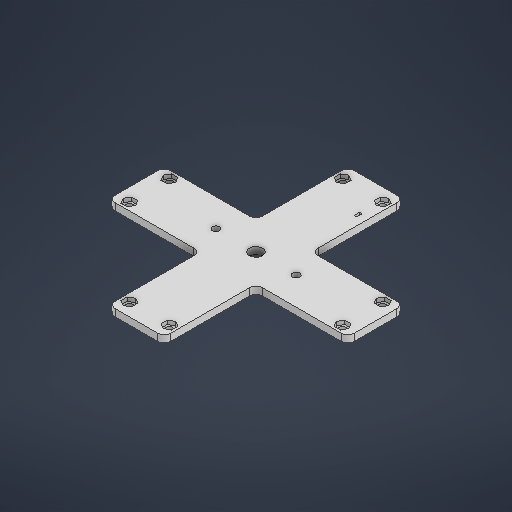
# Autodesk Inventor part: motor_holder
Saved by Autodesk Inventor 2026 (Build 300175050, 175E)
## iProperties
Created: 2025-01-16
Part Number: motor_holder
Material: Generic
Document SubType Name: Modeling
Designer: aduwa
Density: 1 g/cm^3
Appearance: Default
Author: aduwa
Autodesk Inventor part; units mm, degrees
ref_plane "YZ Plane" through (0, 0, 0) normal (1, 0, 0) x (0, 1, 0)
ref_plane "XZ Plane" through (0, 0, 0) normal (0, 1, 0) x (-1, 0, 0)
ref_plane "XY Plane" through (0, 0, 0) normal (0, 0, 1) x (1, 0, 0)
sketch "Sketch1" plane through (0, 0, 0) normal (0, 1, 0) x (1, 0, 0)
  circle A0 centre (0, 0) radius 2.25
  circle A1 centre (31, 0) radius 2.25
  circle A2 centre (0, 31) radius 2.25
  circle A3 centre (31, 31) radius 2.25
  circle A4 centre (15.5, 15.5) radius 5.125
  line L0 (-6, 37) -> (37, 37)
  line L1 (37, 37) -> (37, -6)
  line L2 (37, -6) -> (-6, -6)
  line L3 (-6, -6) -> (-6, 37)
  line L4 (-6, 37) -> (37, -6) construction
  line L5 (37, 37) -> (-6, -6) construction
  line L6 (-6, -6) -> (37, -6)
  circle A5 centre (0, 98) radius 2.75
  circle A6 centre (31, 98) radius 2.75
  line L7 (-6, 37) -> (37, 37)
  line L8 (37, 37) -> (37, 108)
  line L9 (37, 108) -> (-6, 108)
  line L10 (-6, 108) -> (-6, 37)
  line L11 (15.5, 15.5) -> (22.827, 15.5)
  line L12 (13, 103) -> (18, 103)
  line L13 (15.5, 103) -> (15.5, 96.4439)
  arc A7 (0, 95.25) -> (0, 100.75) centre (0, 98) ccw
  circle A8 centre (-15.5, 15.5) radius 2.7971
  circle A9 centre (46.5, 15.5) radius 2.7971
  line L14 (0, 93.4736) -> (-3.92, 95.7368)
  line L15 (-3.92, 95.7368) -> (-3.92, 100.2632)
  line L16 (-3.92, 100.2632) -> (0, 102.5264)
  line L17 (0, 102.5264) -> (3.92, 100.2632)
  line L18 (3.92, 100.2632) -> (3.92, 95.7368)
  line L19 (3.92, 95.7368) -> (0, 93.4736)
  line L20 (4.17, 100.4076) -> (0, 102.8151)
  line L21 (0, 102.8151) -> (-4.17, 100.4076)
  line L22 (-4.17, 100.4076) -> (-4.17, 95.5924)
  line L23 (-4.17, 95.5924) -> (0, 93.1849)
  line L24 (0, 93.1849) -> (4.17, 95.5924)
  line L25 (4.17, 95.5924) -> (4.17, 100.4076)
  circle A10 centre (31, 98) radius 2.75
  circle A11 centre (31, 98) radius 2.75
  arc A12 (31, 100.75) -> (31, 95.25) centre (31, 98) ccw
  line L26 (31, 93.4736) -> (34.92, 95.7368)
  line L27 (34.92, 95.7368) -> (34.92, 100.2632)
  line L28 (34.92, 100.2632) -> (31, 102.5264)
  line L29 (31, 102.5264) -> (27.08, 100.2632)
  line L30 (27.08, 100.2632) -> (27.08, 95.7368)
  line L31 (27.08, 95.7368) -> (31, 93.4736)
  line L32 (26.83, 100.4076) -> (31, 102.8151)
  line L33 (31, 102.8151) -> (35.17, 100.4076)
  line L34 (35.17, 100.4076) -> (35.17, 95.5924)
  line L35 (35.17, 95.5924) -> (31, 93.1849)
  line L36 (31, 93.1849) -> (26.83, 95.5924)
  line L37 (26.83, 95.5924) -> (26.83, 100.4076)
  line L38 (-64.7368, -3.92) -> (-69.2632, -3.92)
  line L39 (-69.4076, -4.17) -> (-64.5924, -4.17)
  line L40 (-69.2632, -3.92) -> (-71.5264, 0)
  line L41 (-71.8151, 0) -> (-69.4076, -4.17)
  circle A13 centre (-67, 31) radius 2.75
  line L42 (-72, 13) -> (-72, 18)
  line L43 (-69.2632, 27.08) -> (-64.7368, 27.08)
  line L44 (-64.7368, 34.92) -> (-69.2632, 34.92)
  line L45 (-64.5924, 26.83) -> (-69.4076, 26.83)
  circle A14 centre (-67, 31) radius 2.75
  circle A15 centre (-67, 31) radius 2.75
  arc A16 (-69.75, 31) -> (-64.25, 31) centre (-67, 31) ccw
  line L46 (-72, 15.5) -> (-65.4439, 15.5)
  line L47 (-69.2632, 34.92) -> (-71.5264, 31)
  line L48 (-71.8151, 31) -> (-69.4076, 35.17)
  line L49 (-69.4076, 35.17) -> (-64.5924, 35.17)
  line L50 (-71.5264, 31) -> (-69.2632, 27.08)
  line L51 (-69.4076, 26.83) -> (-71.8151, 31)
  line L52 (-62.4736, 0) -> (-64.7368, -3.92)
  line L53 (-64.5924, -4.17) -> (-62.1849, 0)
  circle A17 centre (-67, 0) radius 2.75
  arc A18 (-64.25, 0) -> (-69.75, 0) centre (-67, 0) ccw
  line L54 (-71.5264, 0) -> (-69.2632, 3.92)
  line L55 (-69.4076, 4.17) -> (-71.8151, 0)
  line L56 (-69.2632, 3.92) -> (-64.7368, 3.92)
  line L57 (-64.5924, 4.17) -> (-69.4076, 4.17)
  line L58 (-62.1849, 0) -> (-64.5924, 4.17)
  line L59 (-64.7368, 3.92) -> (-62.4736, 0)
  line L60 (-62.1849, 31) -> (-64.5924, 26.83)
  line L61 (-64.7368, 27.08) -> (-62.4736, 31)
  line L62 (-77, -6) -> (-6, -6)
  line L63 (-62.4736, 31) -> (-64.7368, 34.92)
  line L64 (-64.5924, 35.17) -> (-62.1849, 31)
  line L65 (-77, 37) -> (-77, -6)
  line L66 (-6, 37) -> (-77, 37)
  line L67 (34.92, -64.7368) -> (34.92, -69.2632)
  line L68 (35.17, -69.4076) -> (35.17, -64.5924)
  line L69 (34.92, -69.2632) -> (31, -71.5264)
  line L70 (31, -71.8151) -> (35.17, -69.4076)
  circle A19 centre (0, -67) radius 2.75
  line L71 (18, -72) -> (13, -72)
  line L72 (3.92, -69.2632) -> (3.92, -64.7368)
  line L73 (-3.92, -64.7368) -> (-3.92, -69.2632)
  line L74 (4.17, -64.5924) -> (4.17, -69.4076)
  circle A20 centre (0, -67) radius 2.75
  circle A21 centre (0, -67) radius 2.75
  arc A22 (0, -69.75) -> (0, -64.25) centre (0, -67) ccw
  line L75 (15.5, -72) -> (15.5, -65.4439)
  line L76 (-3.92, -69.2632) -> (0, -71.5264)
  line L77 (0, -71.8151) -> (-4.17, -69.4076)
  line L78 (-4.17, -69.4076) -> (-4.17, -64.5924)
  line L79 (0, -71.5264) -> (3.92, -69.2632)
  line L80 (4.17, -69.4076) -> (0, -71.8151)
  line L81 (31, -62.4736) -> (34.92, -64.7368)
  line L82 (35.17, -64.5924) -> (31, -62.1849)
  circle A23 centre (31, -67) radius 2.75
  arc A24 (31, -64.25) -> (31, -69.75) centre (31, -67) ccw
  line L83 (31, -71.5264) -> (27.08, -69.2632)
  line L84 (26.83, -69.4076) -> (31, -71.8151)
  line L85 (27.08, -69.2632) -> (27.08, -64.7368)
  line L86 (26.83, -64.5924) -> (26.83, -69.4076)
  line L87 (31, -62.1849) -> (26.83, -64.5924)
  line L88 (27.08, -64.7368) -> (31, -62.4736)
  line L89 (0, -62.1849) -> (4.17, -64.5924)
  line L90 (3.92, -64.7368) -> (0, -62.4736)
  line L91 (37, -77) -> (37, -6)
  line L92 (0, -62.4736) -> (-3.92, -64.7368)
  line L93 (-4.17, -64.5924) -> (0, -62.1849)
  line L94 (-6, -77) -> (37, -77)
  line L95 (-6, -6) -> (-6, -77)
  line L96 (95.7368, 34.92) -> (100.2632, 34.92)
  line L97 (100.4076, 35.17) -> (95.5924, 35.17)
  line L98 (100.2632, 34.92) -> (102.5264, 31)
  line L99 (102.8151, 31) -> (100.4076, 35.17)
  circle A25 centre (98, 0) radius 2.75
  line L100 (103, 18) -> (103, 13)
  line L101 (100.2632, 3.92) -> (95.7368, 3.92)
  line L102 (95.7368, -3.92) -> (100.2632, -3.92)
  line L103 (95.5924, 4.17) -> (100.4076, 4.17)
  circle A26 centre (98, 0) radius 2.75
  circle A27 centre (98, 0) radius 2.75
  arc A28 (100.75, 0) -> (95.25, 0) centre (98, 0) ccw
  line L104 (103, 15.5) -> (96.4439, 15.5)
  line L105 (100.2632, -3.92) -> (102.5264, 0)
  line L106 (102.8151, 0) -> (100.4076, -4.17)
  line L107 (100.4076, -4.17) -> (95.5924, -4.17)
  line L108 (102.5264, 0) -> (100.2632, 3.92)
  line L109 (100.4076, 4.17) -> (102.8151, 0)
  line L110 (93.4736, 31) -> (95.7368, 34.92)
  line L111 (95.5924, 35.17) -> (93.1849, 31)
  circle A29 centre (98, 31) radius 2.75
  arc A30 (95.25, 31) -> (100.75, 31) centre (98, 31) ccw
  line L112 (102.5264, 31) -> (100.2632, 27.08)
  line L113 (100.4076, 26.83) -> (102.8151, 31)
  line L114 (100.2632, 27.08) -> (95.7368, 27.08)
  line L115 (95.5924, 26.83) -> (100.4076, 26.83)
  line L116 (93.1849, 31) -> (95.5924, 26.83)
  line L117 (95.7368, 27.08) -> (93.4736, 31)
  line L118 (93.1849, 0) -> (95.5924, 4.17)
  line L119 (95.7368, 3.92) -> (93.4736, 0)
  line L120 (108, 37) -> (37, 37)
  line L121 (93.4736, 0) -> (95.7368, -3.92)
  line L122 (95.5924, -4.17) -> (93.1849, 0)
  line L123 (108, -6) -> (108, 37)
  line L124 (37, -6) -> (108, -6)
  point P0 (37, 37)
  point P1 (37, 37)
  point P2 (-3.5, 98)
  point P3 (34.5, 98)
  point P4 (-67, -3.5)
  point P5 (-67, 34.5)
  point P6 (34.5, -67)
  point P7 (-3.5, -67)
  point P8 (98, 34.5)
  point P9 (98, -3.5)
  point P10 (-6, -6)
  point P11 (-6, -6)
  point P12 (-6, -6)
  point P13 (-6, -6)
  point P14 (-6, -6)
  point P15 (37, 37)
  dimension "d3" = 4.5
  dimension "d5" = 31
  dimension "d6" = 10.25
  dimension "d8" = 43
  dimension "d23" = 5.5
  dimension "d24" = 31
  dimension "d25" = 31
  dimension "d27" = 6
  dimension "d28" = 10
  dimension "d71" = 62
  dimension "d72" = 31
  dimension "d73" = 7.84
  dimension "d74" = 0.25
  dimension "d81" = 82.5
  dimension "d84" = 360
  constraints: 250 end point, 31 centre point, 17 symmetric about line, 16 point on circle, 12 coincident, 6 equal radius, 5 horizontal, 4 parallel, 3 horizontal alignment, 3 midpoint, 2 perpendicular, 2 vertical alignment, 1 point on line, 1 vertical, 341 other
  measures "d3" diameter of A0
  measures "d5" distance of A0.centre A2.centre
  measures "d6" diameter of A4
  measures "d8" distance of L0.end L1.end
  measures "d23" diameter of A5
  measures "d24" distance of A6.centre A5.centre
  measures "d25" distance of A1.centre A0.centre
  measures "d27" distance from line of L0 A2.centre
  measures "d28" distance from line of L9 A5.centre
  measures "d71" distance of A9.centre A8.centre
  measures "d72" distance of L11.start A8.centre
  measures "d73" distance between parallel lines of L15 L18
  measures "d74" distance between parallel lines of L17 L20
  measures "d81" vertical distance of L11.start A5.centre
extrude "Extrusion4" add sketch "Sketch1" against normal blind 5.5 contours A0 | A1 | A2 | A3 | L10 L9 L8 L0 | L0 L1 L2 L3 | L3 L62 L65 L66 | L120 L123 L124 L1 | L2 L91 L94 L95 | L14 L15 L16 L17 L18 L19 | L25 L24 L23 L22 L21 L20 | L31 L30 L29 L28 L27 L26 | L32 L33 L34 L35 L36 L37 | L38 L40 L54 L56 L59 L52 | L41 L55 L57 L58 L53 L39 | L50 L47 L44 L63 L61 L43 | L45 L51 L48 L49 L64 L60 | L67 L69 L83 L85 L88 L81 | L70 L84 L86 L87 L82 L68 | L79 L76 L73 L92 L90 L72 | L74 L80 L77 L78 L93 L89 | L96 L98 L112 L114 L117 L110 | L99 L113 L115 L116 L111 L97 | L108 L105 L102 L121 L119 L101 | L103 L109 L106 L107 L122 L118
fillet "Fillet4" radius 5 4 edges at (-6, -2.75, -37) (-6, -2.75, 6) (37, -2.75, 6) (37, -2.75, -37)
fillet "Fillet5" radius 5 8 edges at (37, -2.75, -108) (-6, -2.75, -108) (108, -2.75, 6) (108, -2.75, -37) (37, -2.75, 77) (-6, -2.75, 77) (-77, -2.75, 6) (-77, -2.75, -37)
extrude "Extrusion7" cut sketch "Sketch1" against normal blind 3 contours A5 | A6 | L14 L15 L16 L17 L18 L19 | L25 L24 L23 L22 L21 L20 | L31 L30 L29 L28 L27 L26 | L32 L33 L34 L35 L36 L37 | L38 L40 L54 L56 L59 L52 | L41 L55 L57 L58 L53 L39 | A13 | L50 L47 L44 L63 L61 L43 | L45 L51 L48 L49 L64 L60 | A17 | L67 L69 L83 L85 L88 L81 | L70 L84 L86 L87 L82 L68 | A19 | L79 L76 L73 L92 L90 L72 | L74 L80 L77 L78 L93 L89 | A23 | L96 L98 L112 L114 L117 L110 | L99 L113 L115 L116 L111 L97 | A25 | L108 L105 L102 L121 L119 L101 | L103 L109 L106 L107 L122 L118 | A29
sketch "Sketch6" plane through (0, 0, 0) normal (0, 1, 0) x (1, 0, 0)
  line L0 (31, 78) -> (29, 78)
  line L1 (29, 78) -> (29, 82)
  line L2 (29, 82) -> (31, 82)
  line L3 (31, 82) -> (31, 78)
  line L4 (37, 42) -> (37, 103) projected
  line L5 (32, 108) -> (-1, 108) projected
  circle A0 centre (31, 98) radius 2.75 projected
  point P0 (0, 0)
  dimension "d86" = 2
  dimension "d87" = 4
  dimension "d88" = 6
  dimension "d92" = 16
  constraints: 8 end point, 2 parallel, 1 horizontal, 1 perpendicular
  measures "d86" distance of L1.end L2.end
  measures "d87" distance of L0.end L1.end
  measures "d88" distance between parallel lines of L4 L3
  measures "d92" distance from line of L2 A0.centre
extrude "Extrusion8" cut sketch "Sketch6" against normal through all contours L0 L1 L2 L3
body "Solid2"
